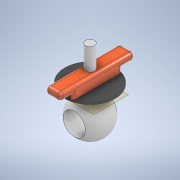
# Autodesk Inventor part: Ventilregler
Saved by Autodesk Inventor 2021 (Build 250183000, 183)
## iProperties
Created: 2021-06-23
Part Number: Ventilregler
Material: Generisch
Document SubType Name: Modeling
Designer: stroh
Density: 1 g/cm^3
Appearance: Vorgabe
Author: stroh
Autodesk Inventor part; units mm, degrees
ref_plane "YZ Plane" through (0, 0, 0) normal (1, 0, 0) x (0, 1, 0)
ref_plane "XY Plane" through (0, 0, 0) normal (0, 0, 1) x (1, 0, 0)
sketch "Skizze1" plane through (0, 0, 0) normal (0, 0, 1) x (1, 0, 0)
  circle A0 centre (0, 0) radius 13
  line L0 (-18.2, 0) -> (18.2, 0) projected
  line L1 (0, -18.2) -> (0, 18.2) projected
  point P0 (0, 13)
  point P1 (0, -13)
  dimension "d0" = 26
  constraints: 1 centre point, 1 coincident
  measures "d0" diameter of A0
revolve "Umdrehung1" add sketch "Skizze1" angle 360 about axis through (0, -10, 0) along (0, 1, 0) picked at (4.582, 7.2921) picked at (8.558, -0.9643) contours L0 L1 A0 | A0 L1 L0
sketch "Skizze2" plane through (0, 0, 0) normal (0, 0, 1) x (1, 0, 0)
  circle A0 centre (0, 0) radius 7.5
  dimension "d2" = 15
  constraints: 1 centre point, 1 coincident
  measures "d2" diameter of A0
extrude "Extrusion1" cut sketch "Skizze2" along normal mid plane 26
ref_plane "Arbeitsebene1" through (0, 13, 0) normal (0, 1, 0) x (-1, 0, 0)
sketch "Skizze3" plane through (0, 13, 0) normal (0, 1, 0) x (-1, 0, 0)
  circle A0 centre (0, 0) radius 5
  dimension "d6" = 10
  constraints: 1 centre point, 1 coincident
  measures "d6" diameter of A0
extrude "Extrusion2" add sketch "Skizze3" along normal blind 5 and the other way blind 1
sketch "Skizze4" plane through (0, 18, 0) normal (0, 1, 0) x (1, 0, 0)
  circle A0 centre (0, 0) radius 17
  dimension "d11" = 34
  constraints: 1 centre point, 1 coincident
  measures "d11" diameter of A0
extrude "Extrusion3" add sketch "Skizze4" along normal blind 1
sketch "Skizze5" plane through (0, 19, 0) normal (0, 1, 0) x (1, 0, 0)
  circle A0 centre (0, 0) radius 17 projected
  line L0 (5, 15.9474) -> (5, -15.9474)
  line L1 (7.5, 10.6184) -> (7.5, -10.6184) projected
  line L2 (5, 15.9474) -> (5, 16.2481)
  line L3 (5, -15.9474) -> (5, -16.2481)
  line L4 (-5, 16.2481) -> (-5, -16.2481)
  arc A1 (-5, -16.2481) -> (5, -16.2481) centre (0, 0) ccw
  arc A2 (5, 16.2481) -> (-5, 16.2481) centre (0, 0) ccw
  dimension "d15" = 5
  dimension "d16" = 5
  constraints: 8 end point, 8 point on circle, 2 centre point, 2 vertical, 1 coincident, 1 parallel, 1 point on line
  measures "d15" distance from line of point (0, 0) L0
  measures "d16" distance from line of point (0, 0) L4
extrude "Extrusion4" add sketch "Skizze5" along normal blind 3 contours L2 L0 L3 A0 L4
sketch "Skizze6" plane through (0, 22, 0) normal (0, 1, 0) x (1, 0, 0)
  line L0 (-5, 25) -> (5, 25)
  line L1 (5, 25) -> (5, -25)
  line L2 (5, -25) -> (-5, -25)
  line L3 (-5, -25) -> (-5, 25)
  line L4 (5, -16.2481) -> (5, 16.2481) projected
  point P0 (0, 0)
  dimension "d19" = 10
  dimension "d20" = 50
  dimension "d21" = 0
  dimension "d22" = 25
  constraints: 8 end point, 2 parallel, 1 horizontal, 1 perpendicular
  measures "d19" distance between parallel lines of L1 L3
  measures "d20" distance between parallel lines of L2 L0
  measures "d21" distance between parallel lines of L4 L1
  measures "d22" distance from line of point (0, 0) L0
extrude "Extrusion5" add sketch "Skizze6" along normal blind 5
fillet "Rundung1" radius 2 18 edges at (0, 27, 25) (0, 22, 25) (5, 24.5, 25) (-5, 24.5, 25) (5, 27, 0) (-5, 27, 0) (5, 22, 20.624) (5, 20.5, 16.2481) (5, 22, -20.624) (5, 20.5, -16.2481) (-5, 22, 20.624) (-5, 20.5, 16.2481) (-5, 20.5, -16.2481) (-5, 22, -20.624) (-5, 24.5, -25) (0, 27, -25) (0, 22, -25) (5, 24.5, -25)
sketch "Skizze7" plane through (0, 27, 0) normal (0, 1, 0) x (1, 0, 0)
  circle A0 centre (0, 0) radius 3
  dimension "d26" = 6
  constraints: 1 centre point, 1 coincident
  measures "d26" diameter of A0
extrude "Extrusion6" add sketch "Skizze7" along normal blind 15
